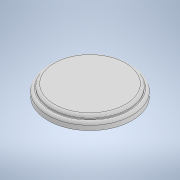
# Autodesk Inventor part: Chess Piece Base
Saved by Autodesk Inventor 2022 (Build 260153000, 153)
## iProperties
Created: 2022-04-22
Part Number: Chess Piece Base
Material: Generic
Document SubType Name: Modeling
Designer: Nick
Density: 1 g/cm^3
Appearance: Default
Author: Nick
Autodesk Inventor part; units mm, degrees
ref_plane "YZ Plane" through (0, 0, 0) normal (1, 0, 0) x (0, 1, 0)
ref_plane "XZ Plane" through (0, 0, 0) normal (0, 1, 0) x (-1, 0, 0)
ref_plane "XY Plane" through (0, 0, 0) normal (0, 0, 1) x (1, 0, 0)
sketch "Sketch1" plane through (0, 0, 0) normal (0, 0, 1) x (1, 0, 0)
  line L0 (0, 0) -> (0, 19.8394)
  line L1 (0, 0) -> (11.5, 0)
  line L2 (11.5, 0) -> (11.5, 2)
  line L3 (11.5, 2) -> (10.5, 2)
  line L4 (10.5, 2) -> (10.5, 3)
  line L5 (10.5, 3) -> (0, 3)
  dimension "d1" = 2
  dimension "d2" = 1
  dimension "d3" = 1
  dimension "d6" = 23
  constraints: 12 end point, 4 perpendicular, 1 horizontal, 1 point on line, 1 vertical
  measures "d1" distance of L1.end L2.end
  measures "d2" distance of L3.end L4.end
  measures "d3" distance of L2.end L3.end
  measures "d6" diameter of L2 L0
revolve "Revolution1" add sketch "Sketch1" angle 360 about axis through (0, 0, 0) along (0, 1, 0)
fillet "Fillet1" radius 0.75 2 edges at (-11.5, 2, 0) (-10.5, 3, 0)
body "Solid1"
